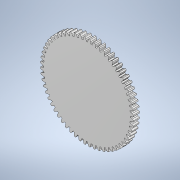
# Autodesk Inventor part: 二段m1z60
Saved by Autodesk Inventor 2022.2 (Build 262287010, 287A)
## iProperties
Created: 2022-03-13
Part Number: 二段m1z60
Material: Aluminum 2014-T6
Document SubType Name: Modeling
Designer: acps
Density: 2.78927 g/cm^3
Appearance: Satin
Author: acps
Autodesk Inventor part; units mm, degrees
ref_plane "YZ Plane" through (0, 0, 0) normal (1, 0, 0) x (0, 1, 0)
ref_plane "XZ Plane" through (0, 0, 0) normal (0, 1, 0) x (-1, 0, 0)
ref_plane "XY Plane" through (0, 0, 0) normal (0, 0, 1) x (1, 0, 0)
sketch "Sketch1" plane through (0, 0, 0) normal (0, 0, 1) x (1, 0, 0)
  arc A0 (0.5381, 29.2813) -> (0.3992, 28.7472) centre (7.046, 27.304) ccw
  arc A1 (0.7944, 30.0128) -> (0.5381, 29.2813) centre (9.2841, 26.6271) ccw
  arc A2 (1.223, 30.9617) -> (0.7944, 30.0128) centre (11.5695, 25.7177) ccw
  arc A3 (-2.5272, 29.1688) -> (-2.6079, 28.6315) centre (4.1534, 27.891) ccw
  arc A4 (-2.3471, 29.9314) -> (-2.5272, 29.1688) centre (6.45, 27.4517) ccw
  arc A5 (-2.0201, 30.9199) -> (-2.3471, 29.9314) centre (8.8179, 26.7861) ccw
  arc A6 (-5.5616, 28.7533) -> (-5.5864, 28.202) centre (1.2152, 28.1723) ccw
  arc A7 (-5.4629, 29.5221) -> (-5.5616, 28.7533) centre (3.5452, 27.9755) ccw
  arc A8 (-5.241, 30.5394) -> (-5.4629, 29.5221) centre (5.9697, 27.5611) ccw
  arc A9 (-8.5367, 28.0144) -> (-8.5037, 27.4636) centre (-1.7362, 28.145) ccw
  arc A10 (-8.5189, 28.7893) -> (-8.5367, 28.0144) centre (0.6015, 28.1928) ccw
  arc A11 (-8.4046, 29.8243) -> (-8.5189, 28.7893) centre (3.0561, 28.0342) ccw
  arc A12 (-11.4182, 26.9686) -> (-11.3278, 26.4243) centre (-4.6687, 27.8093) ccw
  arc A13 (-11.4816, 27.7412) -> (-11.4182, 26.9686) centre (-2.3488, 28.1012) ccw
  arc A14 (-11.476, 28.7824) -> (-11.4816, 27.7412) centre (0.109, 28.2) ccw
  arc A15 (-14.1746, 25.6274) -> (-14.0279, 25.0954) centre (-7.55, 27.169) ccw
  arc A16 (-14.3184, 26.389) -> (-14.1746, 25.6274) centre (-5.2733, 27.7018) ccw
  arc A17 (-14.4217, 27.4251) -> (-14.3184, 26.389) centre (-2.8393, 28.057) ccw
  arc A18 (-16.7758, 24.0053) -> (-16.5742, 23.4917) centre (-10.3486, 26.231) ccw
  arc A19 (-16.9984, 24.7478) -> (-16.7758, 24.0053) centre (-8.14, 26.9988) ccw
  arc A20 (-17.2094, 25.7674) -> (-16.9984, 24.7478) centre (-5.7565, 27.6065) ccw
  arc A21 (-19.1931, 22.1203) -> (-18.939, 21.6305) centre (-13.0337, 25.0056) ccw
  arc A22 (-19.4921, 22.8354) -> (-19.1931, 22.1203) centre (-10.9176, 26.0001) ccw
  arc A23 (-19.8086, 23.8274) -> (-19.4921, 22.8354) centre (-8.6106, 26.8535) ccw
  arc A24 (-21.4002, 19.9929) -> (-21.0962, 19.5323) centre (-15.5761, 23.5062) ccw
  arc A25 (-21.7723, 20.6728) -> (-21.4002, 19.9929) centre (-13.5755, 24.7164) ccw
  arc A26 (-22.1907, 21.6263) -> (-21.7723, 20.6728) centre (-11.3704, 25.8063) ccw
  arc A27 (-23.3728, 17.6464) -> (-23.0223, 17.2202) centre (-17.9479, 21.7493) ccw
  arc A28 (-23.8139, 18.2838) -> (-23.3728, 17.6464) centre (-16.0847, 23.162) ccw
  arc A29 (-24.3297, 19.1883) -> (-23.8139, 18.2838) centre (-14.0056, 24.4764) ccw
  arc A30 (-25.0893, 15.1066) -> (-24.6962, 14.7194) centre (-20.123, 19.754) ccw
  arc A31 (-25.5946, 15.6944) -> (-25.0893, 15.1066) centre (-18.4177, 21.3538) ccw
  arc A32 (-26.2021, 16.54) -> (-25.5946, 15.6944) centre (-16.4874, 22.8784) ccw
  arc A33 (-26.5309, 12.4013) -> (-26.0995, 12.0573) centre (-22.0776, 17.5424) ccw
  arc A34 (-27.0949, 12.933) -> (-26.5309, 12.4013) centre (-20.5489, 19.3117) ccw
  arc A35 (-27.7875, 13.7105) -> (-27.0949, 12.933) centre (-18.7885, 21.0296) ccw
  arc A36 (-27.6819, 9.5602) -> (-27.2169, 9.2631) centre (-23.7903, 15.1386) ccw
  arc A37 (-28.2984, 10.03) -> (-27.6819, 9.5602) centre (-22.4549, 17.0579) ccw
  arc A38 (-29.0684, 10.7308) -> (-28.2984, 10.03) centre (-20.8838, 18.9505) ccw
  arc A39 (-28.5295, 6.6143) -> (-28.036, 6.3674) centre (-25.2424, 12.5689) ccw
  arc A40 (-29.1918, 7.0171) -> (-28.5295, 6.6143) centre (-24.1149, 14.6173) ccw
  arc A41 (-30.0309, 7.6336) -> (-29.1918, 7.0171) centre (-22.7503, 16.6637) ccw
  arc A42 (-29.0646, 3.5959) -> (-28.548, 3.4019) centre (-26.4179, 9.8615) ccw
  arc A43 (-29.7653, 3.9273) -> (-29.0646, 3.5959) centre (-25.5108, 12.0165) ccw
  arc A44 (-30.6643, 4.4527) -> (-29.7653, 3.9273) centre (-24.3675, 14.1944) ccw
  arc A45 (-29.2813, 0.5381) -> (-28.7472, 0.3992) centre (-27.304, 7.046) ccw
  arc A46 (-30.0128, 0.7944) -> (-29.2813, 0.5381) centre (-26.6271, 9.2841) ccw
  arc A47 (-30.9617, 1.223) -> (-30.0128, 0.7944) centre (-25.7177, 11.5695) ccw
  arc A48 (-29.1771, -2.5256) -> (-28.6315, -2.6079) centre (-27.891, 4.1534) ccw
  arc A49 (-29.9314, -2.3471) -> (-29.1771, -2.5256) centre (-27.4517, 6.45) ccw
  arc A50 (-30.9199, -2.0201) -> (-29.9314, -2.3471) centre (-26.7862, 8.8179) ccw
  arc A51 (-28.7533, -5.5616) -> (-28.202, -5.5864) centre (-28.1723, 1.2152) ccw
  arc A52 (-29.5221, -5.4629) -> (-28.7533, -5.5616) centre (-27.9755, 3.5452) ccw
  arc A53 (-30.5394, -5.241) -> (-29.5221, -5.4629) centre (-27.5611, 5.9697) ccw
  arc A54 (-28.0144, -8.5367) -> (-27.4636, -8.5037) centre (-28.145, -1.7362) ccw
  arc A55 (-28.7893, -8.5189) -> (-28.0144, -8.5367) centre (-28.1928, 0.6015) ccw
  arc A56 (-29.8243, -8.4046) -> (-28.7893, -8.5189) centre (-28.0342, 3.0561) ccw
  arc A57 (-26.9686, -11.4182) -> (-26.4243, -11.3278) centre (-27.8093, -4.6687) ccw
  arc A58 (-27.7412, -11.4816) -> (-26.9686, -11.4182) centre (-28.1012, -2.3488) ccw
  arc A59 (-28.7824, -11.476) -> (-27.7412, -11.4816) centre (-28.2, 0.109) ccw
  arc A60 (-25.6274, -14.1746) -> (-25.0954, -14.0279) centre (-27.169, -7.55) ccw
  arc A61 (-26.389, -14.3184) -> (-25.6274, -14.1746) centre (-27.7018, -5.2733) ccw
  arc A62 (-27.4251, -14.4217) -> (-26.389, -14.3184) centre (-28.057, -2.8393) ccw
  arc A63 (-24.0053, -16.7758) -> (-23.4917, -16.5742) centre (-26.231, -10.3486) ccw
  arc A64 (-24.741, -16.9966) -> (-24.0053, -16.7758) centre (-26.9988, -8.14) ccw
  arc A65 (-25.7674, -17.2094) -> (-24.741, -16.9966) centre (-27.6065, -5.7565) ccw
  arc A66 (-22.1126, -19.1895) -> (-21.6305, -18.939) centre (-25.0056, -13.0337) ccw
  arc A67 (-22.8354, -19.4921) -> (-22.1126, -19.1895) centre (-26.0001, -10.9176) ccw
  arc A68 (-23.8274, -19.8086) -> (-22.8354, -19.4921) centre (-26.8535, -8.6106) ccw
  arc A69 (-19.9929, -21.4002) -> (-19.5323, -21.0962) centre (-23.5062, -15.5761) ccw
  arc A70 (-20.6728, -21.7723) -> (-19.9929, -21.4002) centre (-24.7164, -13.5755) ccw
  arc A71 (-21.6263, -22.1907) -> (-20.6728, -21.7723) centre (-25.8063, -11.3704) ccw
  arc A72 (-17.6464, -23.3728) -> (-17.2202, -23.0223) centre (-21.7493, -17.9479) ccw
  arc A73 (-18.2838, -23.8139) -> (-17.6464, -23.3728) centre (-23.162, -16.0847) ccw
  arc A74 (-19.1883, -24.3297) -> (-18.2838, -23.8139) centre (-24.4764, -14.0056) ccw
  arc A75 (-15.1066, -25.0893) -> (-14.7194, -24.6962) centre (-19.754, -20.123) ccw
  arc A76 (-15.6944, -25.5946) -> (-15.1066, -25.0893) centre (-21.3538, -18.4177) ccw
  arc A77 (-16.54, -26.2021) -> (-15.6944, -25.5946) centre (-22.8784, -16.4874) ccw
  arc A78 (-12.4013, -26.5309) -> (-12.0573, -26.0995) centre (-17.5424, -22.0776) ccw
  arc A79 (-12.933, -27.0949) -> (-12.4013, -26.5309) centre (-19.3117, -20.5489) ccw
  arc A80 (-13.7105, -27.7875) -> (-12.933, -27.0949) centre (-21.0296, -18.7885) ccw
  arc A81 (-9.5602, -27.6819) -> (-9.2631, -27.2169) centre (-15.1386, -23.7903) ccw
  arc A82 (-10.03, -28.2984) -> (-9.5602, -27.6819) centre (-17.0579, -22.4549) ccw
  arc A83 (-10.7308, -29.0684) -> (-10.03, -28.2984) centre (-18.9505, -20.8838) ccw
  arc A84 (-6.6143, -28.5295) -> (-6.3674, -28.036) centre (-12.5689, -25.2424) ccw
  arc A85 (-7.0171, -29.1918) -> (-6.6143, -28.5295) centre (-14.6173, -24.1149) ccw
  arc A86 (-7.6336, -30.0309) -> (-7.0171, -29.1918) centre (-16.6637, -22.7503) ccw
  arc A87 (-3.5959, -29.0646) -> (-3.4019, -28.548) centre (-9.8615, -26.4179) ccw
  arc A88 (-3.9273, -29.7653) -> (-3.5959, -29.0646) centre (-12.0165, -25.5108) ccw
  arc A89 (-4.4527, -30.6643) -> (-3.9273, -29.7653) centre (-14.1944, -24.3675) ccw
  arc A90 (-0.5381, -29.2813) -> (-0.3992, -28.7472) centre (-7.046, -27.304) ccw
  arc A91 (-0.7944, -30.0128) -> (-0.5381, -29.2813) centre (-9.2841, -26.6271) ccw
  arc A92 (-1.223, -30.9617) -> (-0.7944, -30.0128) centre (-11.5695, -25.7177) ccw
  arc A93 (2.5256, -29.1771) -> (2.6079, -28.6315) centre (-4.1534, -27.891) ccw
  arc A94 (2.3471, -29.9314) -> (2.5256, -29.1771) centre (-6.45, -27.4517) ccw
  arc A95 (2.0201, -30.9199) -> (2.3471, -29.9314) centre (-8.8179, -26.7862) ccw
  arc A96 (5.5616, -28.7533) -> (5.5864, -28.202) centre (-1.2152, -28.1723) ccw
  arc A97 (5.4629, -29.5221) -> (5.5616, -28.7533) centre (-3.5452, -27.9755) ccw
  arc A98 (5.241, -30.5394) -> (5.4629, -29.5221) centre (-5.9697, -27.5611) ccw
  arc A99 (8.5367, -28.0144) -> (8.5037, -27.4636) centre (1.7362, -28.145) ccw
  arc A100 (8.5189, -28.7893) -> (8.5367, -28.0144) centre (-0.6015, -28.1928) ccw
  arc A101 (8.4046, -29.8243) -> (8.5189, -28.7893) centre (-3.0561, -28.0342) ccw
  arc A102 (11.4182, -26.9686) -> (11.3278, -26.4243) centre (4.6687, -27.8093) ccw
  arc A103 (11.4816, -27.7412) -> (11.4182, -26.9686) centre (2.3488, -28.1012) ccw
  arc A104 (11.476, -28.7824) -> (11.4816, -27.7412) centre (-0.109, -28.2) ccw
  arc A105 (14.1746, -25.6274) -> (14.0279, -25.0954) centre (7.55, -27.169) ccw
  arc A106 (14.3184, -26.389) -> (14.1746, -25.6274) centre (5.2733, -27.7018) ccw
  arc A107 (14.4217, -27.4251) -> (14.3184, -26.389) centre (2.8393, -28.057) ccw
  arc A108 (16.7758, -24.0053) -> (16.5742, -23.4917) centre (10.3486, -26.231) ccw
  arc A109 (16.9984, -24.7478) -> (16.7758, -24.0053) centre (8.14, -26.9988) ccw
  arc A110 (17.2094, -25.7674) -> (16.9984, -24.7478) centre (5.7565, -27.6065) ccw
  arc A111 (19.1931, -22.1203) -> (18.939, -21.6305) centre (13.0337, -25.0056) ccw
  arc A112 (19.4921, -22.8354) -> (19.1931, -22.1203) centre (10.9176, -26.0001) ccw
  arc A113 (19.8086, -23.8274) -> (19.4921, -22.8354) centre (8.6106, -26.8535) ccw
  arc A114 (21.4002, -19.9929) -> (21.0962, -19.5323) centre (15.5761, -23.5062) ccw
  arc A115 (21.7723, -20.6728) -> (21.4002, -19.9929) centre (13.5755, -24.7164) ccw
  arc A116 (22.1907, -21.6263) -> (21.7723, -20.6728) centre (11.3704, -25.8063) ccw
  arc A117 (23.3728, -17.6464) -> (23.0223, -17.2202) centre (17.9479, -21.7493) ccw
  arc A118 (23.8139, -18.2838) -> (23.3728, -17.6464) centre (16.0847, -23.162) ccw
  arc A119 (24.3297, -19.1883) -> (23.8139, -18.2838) centre (14.0056, -24.4764) ccw
  arc A120 (25.0893, -15.1066) -> (24.6962, -14.7194) centre (20.123, -19.754) ccw
  arc A121 (25.5946, -15.6944) -> (25.0893, -15.1066) centre (18.4177, -21.3538) ccw
  arc A122 (26.2021, -16.54) -> (25.5946, -15.6944) centre (16.4874, -22.8784) ccw
  arc A123 (26.5309, -12.4013) -> (26.0995, -12.0573) centre (22.0776, -17.5424) ccw
  arc A124 (27.0949, -12.933) -> (26.5309, -12.4013) centre (20.5489, -19.3117) ccw
  arc A125 (27.7875, -13.7105) -> (27.0949, -12.933) centre (18.7885, -21.0296) ccw
  arc A126 (27.6819, -9.5602) -> (27.2169, -9.2631) centre (23.7903, -15.1386) ccw
  arc A127 (28.2984, -10.03) -> (27.6819, -9.5602) centre (22.4549, -17.0579) ccw
  arc A128 (29.0684, -10.7308) -> (28.2984, -10.03) centre (20.8838, -18.9505) ccw
  arc A129 (28.5295, -6.6143) -> (28.036, -6.3674) centre (25.2424, -12.5689) ccw
  arc A130 (29.1918, -7.0171) -> (28.5295, -6.6143) centre (24.1149, -14.6173) ccw
  arc A131 (30.0309, -7.6336) -> (29.1918, -7.0171) centre (22.7503, -16.6637) ccw
  arc A132 (29.0646, -3.5959) -> (28.548, -3.4019) centre (26.4179, -9.8615) ccw
  arc A133 (29.7653, -3.9273) -> (29.0646, -3.5959) centre (25.5108, -12.0165) ccw
  arc A134 (30.6643, -4.4527) -> (29.7653, -3.9273) centre (24.3675, -14.1944) ccw
  arc A135 (29.2813, -0.5381) -> (28.7472, -0.3992) centre (27.304, -7.046) ccw
  arc A136 (30.0128, -0.7944) -> (29.2813, -0.5381) centre (26.6271, -9.2841) ccw
  arc A137 (30.9617, -1.223) -> (30.0128, -0.7944) centre (25.7177, -11.5695) ccw
  arc A138 (29.1771, 2.5256) -> (28.6315, 2.6079) centre (27.891, -4.1534) ccw
  arc A139 (29.9314, 2.3471) -> (29.1771, 2.5256) centre (27.4517, -6.45) ccw
  arc A140 (30.9199, 2.0201) -> (29.9314, 2.3471) centre (26.7862, -8.8179) ccw
  arc A141 (28.7533, 5.5616) -> (28.202, 5.5864) centre (28.1723, -1.2152) ccw
  arc A142 (29.5221, 5.4629) -> (28.7533, 5.5616) centre (27.9755, -3.5452) ccw
  arc A143 (30.5394, 5.241) -> (29.5221, 5.4629) centre (27.5611, -5.9697) ccw
  arc A144 (28.0144, 8.5367) -> (27.4636, 8.5037) centre (28.145, 1.7362) ccw
  arc A145 (28.7893, 8.5189) -> (28.0144, 8.5367) centre (28.1928, -0.6015) ccw
  arc A146 (29.8243, 8.4046) -> (28.7893, 8.5189) centre (28.0342, -3.0561) ccw
  arc A147 (26.9686, 11.4182) -> (26.4243, 11.3278) centre (27.8093, 4.6687) ccw
  arc A148 (27.7412, 11.4816) -> (26.9686, 11.4182) centre (28.1012, 2.3488) ccw
  arc A149 (28.7824, 11.476) -> (27.7412, 11.4816) centre (28.2, -0.109) ccw
  arc A150 (25.6274, 14.1746) -> (25.0954, 14.0279) centre (27.169, 7.55) ccw
  arc A151 (26.389, 14.3184) -> (25.6274, 14.1746) centre (27.7018, 5.2733) ccw
  arc A152 (27.4251, 14.4217) -> (26.389, 14.3184) centre (28.057, 2.8393) ccw
  arc A153 (24.0053, 16.7758) -> (23.4917, 16.5742) centre (26.231, 10.3486) ccw
  arc A154 (24.7478, 16.9984) -> (24.0053, 16.7758) centre (26.9988, 8.14) ccw
  arc A155 (25.7674, 17.2094) -> (24.7478, 16.9984) centre (27.6065, 5.7565) ccw
  arc A156 (22.1203, 19.1931) -> (21.6305, 18.939) centre (25.0056, 13.0337) ccw
  arc A157 (22.8354, 19.4921) -> (22.1203, 19.1931) centre (26.0001, 10.9176) ccw
  arc A158 (23.8274, 19.8086) -> (22.8354, 19.4921) centre (26.8535, 8.6106) ccw
  arc A159 (19.9929, 21.4002) -> (19.5323, 21.0962) centre (23.5062, 15.5761) ccw
  arc A160 (20.6728, 21.7723) -> (19.9929, 21.4002) centre (24.7164, 13.5755) ccw
  arc A161 (21.6263, 22.1907) -> (20.6728, 21.7723) centre (25.8063, 11.3704) ccw
  arc A162 (17.6464, 23.3728) -> (17.2202, 23.0223) centre (21.7493, 17.9479) ccw
  arc A163 (18.2838, 23.8139) -> (17.6464, 23.3728) centre (23.162, 16.0847) ccw
  arc A164 (19.1883, 24.3297) -> (18.2838, 23.8139) centre (24.4764, 14.0056) ccw
  arc A165 (15.1066, 25.0893) -> (14.7194, 24.6962) centre (19.754, 20.123) ccw
  arc A166 (15.6944, 25.5946) -> (15.1066, 25.0893) centre (21.3538, 18.4177) ccw
  arc A167 (16.54, 26.2021) -> (15.6944, 25.5946) centre (22.8784, 16.4874) ccw
  arc A168 (12.4013, 26.5309) -> (12.0573, 26.0995) centre (17.5424, 22.0776) ccw
  arc A169 (12.933, 27.0949) -> (12.4013, 26.5309) centre (19.3117, 20.5489) ccw
  arc A170 (13.7105, 27.7875) -> (12.933, 27.0949) centre (21.0296, 18.7885) ccw
  arc A171 (9.5602, 27.6819) -> (9.2631, 27.2169) centre (15.1386, 23.7903) ccw
  arc A172 (10.03, 28.2984) -> (9.5602, 27.6819) centre (17.0579, 22.4549) ccw
  arc A173 (10.7308, 29.0684) -> (10.03, 28.2984) centre (18.9505, 20.8838) ccw
  arc A174 (6.6143, 28.5295) -> (6.3674, 28.036) centre (12.5689, 25.2424) ccw
  arc A175 (7.0171, 29.1918) -> (6.6143, 28.5295) centre (14.6173, 24.1149) ccw
  arc A176 (7.6336, 30.0309) -> (7.0171, 29.1918) centre (16.6637, 22.7503) ccw
  arc A177 (3.5959, 29.0646) -> (3.4019, 28.548) centre (9.8615, 26.4179) ccw
  arc A178 (3.9273, 29.7653) -> (3.5959, 29.0646) centre (12.0165, 25.5108) ccw
  arc A179 (4.4527, 30.6643) -> (3.9273, 29.7653) centre (14.1944, 24.3675) ccw
  arc A180 (-0.3992, 28.7472) -> (-0.5381, 29.2813) centre (-7.046, 27.304) ccw
  arc A181 (-0.5381, 29.2813) -> (-0.7944, 30.0128) centre (-9.2841, 26.6271) ccw
  arc A182 (-0.7944, 30.0128) -> (-1.223, 30.9617) centre (-11.5695, 25.7177) ccw
  arc A183 (-3.4019, 28.548) -> (-3.5959, 29.0646) centre (-9.8615, 26.4179) ccw
  arc A184 (-3.5959, 29.0646) -> (-3.9273, 29.7653) centre (-12.0165, 25.5108) ccw
  arc A185 (-3.9273, 29.7653) -> (-4.4527, 30.6643) centre (-14.1944, 24.3675) ccw
  arc A186 (-6.3674, 28.036) -> (-6.6143, 28.5295) centre (-12.5689, 25.2424) ccw
  arc A187 (-6.6143, 28.5295) -> (-7.0171, 29.1918) centre (-14.6173, 24.1149) ccw
  arc A188 (-7.0171, 29.1918) -> (-7.6336, 30.0309) centre (-16.6637, 22.7503) ccw
  arc A189 (-9.2631, 27.2169) -> (-9.5602, 27.6819) centre (-15.1386, 23.7903) ccw
  arc A190 (-9.5602, 27.6819) -> (-10.03, 28.2984) centre (-17.0579, 22.4549) ccw
  arc A191 (-10.03, 28.2984) -> (-10.7308, 29.0684) centre (-18.9505, 20.8838) ccw
  arc A192 (-12.0573, 26.0995) -> (-12.4013, 26.5309) centre (-17.5424, 22.0776) ccw
  arc A193 (-12.4013, 26.5309) -> (-12.933, 27.0949) centre (-19.3117, 20.5489) ccw
  arc A194 (-12.933, 27.0949) -> (-13.7105, 27.7875) centre (-21.0296, 18.7885) ccw
  arc A195 (-14.7194, 24.6962) -> (-15.1066, 25.0893) centre (-19.754, 20.123) ccw
  arc A196 (-15.1066, 25.0893) -> (-15.6944, 25.5946) centre (-21.3538, 18.4177) ccw
  arc A197 (-15.6944, 25.5946) -> (-16.54, 26.2021) centre (-22.8784, 16.4874) ccw
  arc A198 (-17.2202, 23.0223) -> (-17.6464, 23.3728) centre (-21.7493, 17.9479) ccw
  arc A199 (-17.6464, 23.3728) -> (-18.2838, 23.8139) centre (-23.162, 16.0847) ccw
  arc A200 (-18.2838, 23.8139) -> (-19.1883, 24.3297) centre (-24.4764, 14.0056) ccw
  arc A201 (-19.5323, 21.0962) -> (-19.9929, 21.4002) centre (-23.5062, 15.5761) ccw
  arc A202 (-19.9929, 21.4002) -> (-20.6728, 21.7723) centre (-24.7164, 13.5755) ccw
  arc A203 (-20.6728, 21.7723) -> (-21.6263, 22.1907) centre (-25.8063, 11.3704) ccw
  arc A204 (-21.6305, 18.939) -> (-22.1203, 19.1931) centre (-25.0056, 13.0337) ccw
  arc A205 (-22.1203, 19.1931) -> (-22.8354, 19.4921) centre (-26.0001, 10.9176) ccw
  arc A206 (-22.8354, 19.4921) -> (-23.8274, 19.8086) centre (-26.8535, 8.6106) ccw
  arc A207 (-23.4917, 16.5742) -> (-24.0053, 16.7758) centre (-26.231, 10.3486) ccw
  arc A208 (-24.0053, 16.7758) -> (-24.7478, 16.9984) centre (-26.9988, 8.14) ccw
  arc A209 (-24.7478, 16.9984) -> (-25.7674, 17.2094) centre (-27.6065, 5.7565) ccw
  arc A210 (-25.0954, 14.0279) -> (-25.6274, 14.1746) centre (-27.169, 7.55) ccw
  arc A211 (-25.6274, 14.1746) -> (-26.389, 14.3184) centre (-27.7018, 5.2733) ccw
  arc A212 (-26.389, 14.3184) -> (-27.4251, 14.4217) centre (-28.057, 2.8393) ccw
  arc A213 (-26.4243, 11.3278) -> (-26.9686, 11.4182) centre (-27.8093, 4.6687) ccw
  arc A214 (-26.9686, 11.4182) -> (-27.7412, 11.4816) centre (-28.1012, 2.3488) ccw
  arc A215 (-27.7412, 11.4816) -> (-28.7824, 11.476) centre (-28.2, -0.109) ccw
  arc A216 (-27.4636, 8.5037) -> (-28.0144, 8.5367) centre (-28.145, 1.7362) ccw
  arc A217 (-28.0144, 8.5367) -> (-28.7893, 8.5189) centre (-28.1928, -0.6015) ccw
  arc A218 (-28.7893, 8.5189) -> (-29.8243, 8.4046) centre (-28.0342, -3.0561) ccw
  arc A219 (-28.202, 5.5864) -> (-28.7533, 5.5616) centre (-28.1723, -1.2152) ccw
  arc A220 (-28.7533, 5.5616) -> (-29.5221, 5.4629) centre (-27.9755, -3.5452) ccw
  arc A221 (-29.5221, 5.4629) -> (-30.5394, 5.241) centre (-27.5611, -5.9697) ccw
  arc A222 (-28.6315, 2.6079) -> (-29.1771, 2.5256) centre (-27.891, -4.1534) ccw
  arc A223 (-29.1771, 2.5256) -> (-29.9314, 2.3471) centre (-27.4517, -6.45) ccw
  arc A224 (-29.9314, 2.3471) -> (-30.9199, 2.0201) centre (-26.7862, -8.8179) ccw
  arc A225 (-28.7472, -0.3992) -> (-29.2813, -0.5381) centre (-27.304, -7.046) ccw
  arc A226 (-29.2813, -0.5381) -> (-30.0128, -0.7944) centre (-26.6271, -9.2841) ccw
  arc A227 (-30.0128, -0.7944) -> (-30.9617, -1.223) centre (-25.7177, -11.5695) ccw
  arc A228 (-28.548, -3.4019) -> (-29.0646, -3.5959) centre (-26.4179, -9.8615) ccw
  arc A229 (-29.0646, -3.5959) -> (-29.7653, -3.9273) centre (-25.5108, -12.0165) ccw
  arc A230 (-29.7653, -3.9273) -> (-30.6643, -4.4527) centre (-24.3675, -14.1944) ccw
  arc A231 (-28.036, -6.3674) -> (-28.5295, -6.6143) centre (-25.2424, -12.5689) ccw
  arc A232 (-28.5295, -6.6143) -> (-29.1918, -7.0171) centre (-24.1149, -14.6173) ccw
  arc A233 (-29.1918, -7.0171) -> (-30.0309, -7.6336) centre (-22.7503, -16.6637) ccw
  arc A234 (-27.2169, -9.2631) -> (-27.6819, -9.5602) centre (-23.7903, -15.1386) ccw
  arc A235 (-27.6819, -9.5602) -> (-28.2984, -10.03) centre (-22.4549, -17.0579) ccw
  arc A236 (-28.2984, -10.03) -> (-29.0684, -10.7308) centre (-20.8838, -18.9505) ccw
  arc A237 (-26.0995, -12.0573) -> (-26.5309, -12.4013) centre (-22.0776, -17.5424) ccw
  arc A238 (-26.5309, -12.4013) -> (-27.0949, -12.933) centre (-20.5489, -19.3117) ccw
  arc A239 (-27.0949, -12.933) -> (-27.7875, -13.7105) centre (-18.7885, -21.0296) ccw
  arc A240 (-24.6962, -14.7194) -> (-25.0893, -15.1066) centre (-20.123, -19.754) ccw
  arc A241 (-25.0893, -15.1066) -> (-25.5946, -15.6944) centre (-18.4177, -21.3538) ccw
  arc A242 (-25.5946, -15.6944) -> (-26.2021, -16.54) centre (-16.4874, -22.8784) ccw
  arc A243 (-23.0223, -17.2202) -> (-23.3728, -17.6464) centre (-17.9479, -21.7493) ccw
  arc A244 (-23.3728, -17.6464) -> (-23.8139, -18.2838) centre (-16.0847, -23.162) ccw
  arc A245 (-23.8139, -18.2838) -> (-24.3297, -19.1883) centre (-14.0056, -24.4764) ccw
  arc A246 (-21.0962, -19.5323) -> (-21.4002, -19.9929) centre (-15.5761, -23.5062) ccw
  arc A247 (-21.4002, -19.9929) -> (-21.7723, -20.6728) centre (-13.5755, -24.7164) ccw
  arc A248 (-21.7723, -20.6728) -> (-22.1907, -21.6263) centre (-11.3704, -25.8063) ccw
  arc A249 (-18.939, -21.6305) -> (-19.1931, -22.1203) centre (-13.0337, -25.0056) ccw
  arc A250 (-19.1931, -22.1203) -> (-19.4921, -22.8354) centre (-10.9176, -26.0001) ccw
  arc A251 (-19.4921, -22.8354) -> (-19.8086, -23.8274) centre (-8.6106, -26.8535) ccw
  arc A252 (-16.5742, -23.4917) -> (-16.7758, -24.0053) centre (-10.3486, -26.231) ccw
  arc A253 (-16.7758, -24.0053) -> (-16.9984, -24.7478) centre (-8.14, -26.9988) ccw
  arc A254 (-16.9984, -24.7478) -> (-17.2094, -25.7674) centre (-5.7565, -27.6065) ccw
  arc A255 (-14.0279, -25.0954) -> (-14.1746, -25.6274) centre (-7.55, -27.169) ccw
  arc A256 (-14.1746, -25.6274) -> (-14.3184, -26.389) centre (-5.2733, -27.7018) ccw
  arc A257 (-14.3184, -26.389) -> (-14.4217, -27.4251) centre (-2.8393, -28.0569) ccw
  arc A258 (-11.3278, -26.4243) -> (-11.4182, -26.9686) centre (-4.6687, -27.8093) ccw
  arc A259 (-11.4182, -26.9686) -> (-11.4816, -27.7411) centre (-2.3488, -28.1012) ccw
  arc A260 (-11.4816, -27.7411) -> (-11.476, -28.7824) centre (0.109, -28.2) ccw
  arc A261 (-8.5037, -27.4636) -> (-8.5367, -28.0144) centre (-1.7362, -28.145) ccw
  arc A262 (-8.5367, -28.0144) -> (-8.5189, -28.7893) centre (0.6015, -28.1928) ccw
  arc A263 (-8.5189, -28.7893) -> (-8.4046, -29.8243) centre (3.0561, -28.0342) ccw
  arc A264 (-5.5864, -28.202) -> (-5.5616, -28.7533) centre (1.2152, -28.1723) ccw
  arc A265 (-5.5616, -28.7533) -> (-5.4629, -29.5221) centre (3.5452, -27.9755) ccw
  arc A266 (-5.4629, -29.5221) -> (-5.241, -30.5394) centre (5.9697, -27.5611) ccw
  arc A267 (-2.6079, -28.6315) -> (-2.5256, -29.1771) centre (4.1534, -27.891) ccw
  arc A268 (-2.5256, -29.1771) -> (-2.3471, -29.9314) centre (6.45, -27.4517) ccw
  arc A269 (-2.3471, -29.9314) -> (-2.0201, -30.9199) centre (8.8179, -26.7862) ccw
  arc A270 (0.3992, -28.7472) -> (0.5356, -29.2732) centre (7.046, -27.304) ccw
  arc A271 (0.5356, -29.2732) -> (0.7944, -30.0128) centre (9.2841, -26.6271) ccw
  arc A272 (0.7944, -30.0128) -> (1.223, -30.9617) centre (11.5695, -25.7177) ccw
  arc A273 (3.4019, -28.548) -> (3.5959, -29.0646) centre (9.8615, -26.4179) ccw
  arc A274 (3.5959, -29.0646) -> (3.924, -29.7591) centre (12.0165, -25.5108) ccw
  arc A275 (3.924, -29.7591) -> (4.4527, -30.6643) centre (14.1944, -24.3675) ccw
  arc A276 (6.3674, -28.036) -> (6.6143, -28.5295) centre (12.5689, -25.2424) ccw
  arc A277 (6.6143, -28.5295) -> (7.0171, -29.1918) centre (14.6173, -24.1149) ccw
  arc A278 (7.0171, -29.1918) -> (7.6336, -30.0309) centre (16.6637, -22.7503) ccw
  arc A279 (9.2631, -27.2169) -> (9.5553, -27.6749) centre (15.1386, -23.7903) ccw
  arc A280 (9.5553, -27.6749) -> (10.03, -28.2984) centre (17.0579, -22.4549) ccw
  arc A281 (10.03, -28.2984) -> (10.7308, -29.0684) centre (18.9505, -20.8838) ccw
  arc A282 (12.0573, -26.0995) -> (12.4013, -26.5309) centre (17.5424, -22.0776) ccw
  arc A283 (12.4013, -26.5309) -> (12.933, -27.0949) centre (19.3117, -20.5489) ccw
  arc A284 (12.933, -27.0949) -> (13.7105, -27.7875) centre (21.0296, -18.7885) ccw
  arc A285 (14.7194, -24.6962) -> (15.1066, -25.0893) centre (19.754, -20.123) ccw
  arc A286 (15.1066, -25.0893) -> (15.6944, -25.5946) centre (21.3538, -18.4177) ccw
  arc A287 (15.6944, -25.5946) -> (16.54, -26.2021) centre (22.8784, -16.4874) ccw
  arc A288 (17.2202, -23.0223) -> (17.6464, -23.3728) centre (21.7493, -17.9479) ccw
  arc A289 (17.6464, -23.3728) -> (18.2838, -23.8139) centre (23.162, -16.0847) ccw
  arc A290 (18.2838, -23.8139) -> (19.1883, -24.3297) centre (24.4764, -14.0056) ccw
  arc A291 (19.5323, -21.0962) -> (19.9929, -21.4002) centre (23.5062, -15.5761) ccw
  arc A292 (19.9929, -21.4002) -> (20.6728, -21.7723) centre (24.7164, -13.5755) ccw
  arc A293 (20.6728, -21.7723) -> (21.6263, -22.1907) centre (25.8063, -11.3704) ccw
  arc A294 (21.6305, -18.939) -> (22.1203, -19.1931) centre (25.0056, -13.0337) ccw
  arc A295 (22.1203, -19.1931) -> (22.8354, -19.4921) centre (26.0001, -10.9176) ccw
  arc A296 (22.8354, -19.4921) -> (23.8274, -19.8086) centre (26.8535, -8.6106) ccw
  arc A297 (23.4917, -16.5742) -> (24.0053, -16.7758) centre (26.231, -10.3486) ccw
  arc A298 (24.0053, -16.7758) -> (24.7478, -16.9984) centre (26.9988, -8.14) ccw
  arc A299 (24.7478, -16.9984) -> (25.7674, -17.2094) centre (27.6065, -5.7565) ccw
  arc A300 (25.0954, -14.0279) -> (25.6274, -14.1746) centre (27.169, -7.55) ccw
  arc A301 (25.6274, -14.1746) -> (26.389, -14.3184) centre (27.7018, -5.2733) ccw
  arc A302 (26.389, -14.3184) -> (27.4251, -14.4217) centre (28.057, -2.8393) ccw
  arc A303 (26.4243, -11.3278) -> (26.9686, -11.4182) centre (27.8093, -4.6687) ccw
  arc A304 (26.9686, -11.4182) -> (27.7412, -11.4816) centre (28.1012, -2.3488) ccw
  arc A305 (27.7412, -11.4816) -> (28.7824, -11.476) centre (28.2, 0.109) ccw
  arc A306 (27.4636, -8.5037) -> (28.006, -8.5365) centre (28.145, -1.7362) ccw
  arc A307 (28.006, -8.5365) -> (28.7893, -8.5189) centre (28.1928, 0.6015) ccw
  arc A308 (28.7893, -8.5189) -> (29.8243, -8.4046) centre (28.0342, 3.0561) ccw
  arc A309 (28.202, -5.5864) -> (28.7533, -5.5616) centre (28.1723, 1.2152) ccw
  arc A310 (28.7533, -5.5616) -> (29.5221, -5.4629) centre (27.9755, 3.5452) ccw
  arc A311 (29.5221, -5.4629) -> (30.5394, -5.241) centre (27.5611, 5.9697) ccw
  arc A312 (28.6315, -2.6079) -> (29.1771, -2.5256) centre (27.891, 4.1534) ccw
  arc A313 (29.1771, -2.5256) -> (29.9314, -2.3471) centre (27.4517, 6.45) ccw
  arc A314 (29.9314, -2.3471) -> (30.9199, -2.0201) centre (26.7862, 8.8179) ccw
  arc A315 (28.7472, 0.3992) -> (29.2813, 0.5381) centre (27.304, 7.046) ccw
  arc A316 (29.2813, 0.5381) -> (30.0128, 0.7944) centre (26.6271, 9.2841) ccw
  arc A317 (30.0128, 0.7944) -> (30.9617, 1.223) centre (25.7177, 11.5695) ccw
  arc A318 (28.548, 3.4019) -> (29.0646, 3.5959) centre (26.4179, 9.8615) ccw
  arc A319 (29.0646, 3.5959) -> (29.7653, 3.9273) centre (25.5108, 12.0165) ccw
  arc A320 (29.7653, 3.9273) -> (30.6643, 4.4527) centre (24.3675, 14.1944) ccw
  arc A321 (28.036, 6.3674) -> (28.5295, 6.6143) centre (25.2424, 12.5689) ccw
  arc A322 (28.5295, 6.6143) -> (29.1918, 7.0171) centre (24.1149, 14.6173) ccw
  arc A323 (29.1918, 7.0171) -> (30.0309, 7.6336) centre (22.7503, 16.6637) ccw
  arc A324 (27.2169, 9.2631) -> (27.6819, 9.5602) centre (23.7903, 15.1386) ccw
  arc A325 (27.6819, 9.5602) -> (28.2984, 10.03) centre (22.4549, 17.0579) ccw
  arc A326 (28.2984, 10.03) -> (29.0684, 10.7308) centre (20.8838, 18.9505) ccw
  arc A327 (26.0995, 12.0573) -> (26.5309, 12.4013) centre (22.0776, 17.5424) ccw
  arc A328 (26.5309, 12.4013) -> (27.0949, 12.933) centre (20.5489, 19.3117) ccw
  arc A329 (27.0949, 12.933) -> (27.7875, 13.7105) centre (18.7885, 21.0296) ccw
  arc A330 (24.6962, 14.7194) -> (25.0893, 15.1066) centre (20.123, 19.754) ccw
  arc A331 (25.0893, 15.1066) -> (25.5946, 15.6944) centre (18.4177, 21.3538) ccw
  arc A332 (25.5946, 15.6944) -> (26.2021, 16.54) centre (16.4874, 22.8784) ccw
  arc A333 (23.0223, 17.2202) -> (23.3728, 17.6464) centre (17.9479, 21.7493) ccw
  arc A334 (23.3728, 17.6464) -> (23.8139, 18.2838) centre (16.0847, 23.162) ccw
  arc A335 (23.8139, 18.2838) -> (24.3297, 19.1883) centre (14.0056, 24.4764) ccw
  arc A336 (21.0962, 19.5323) -> (21.4002, 19.9929) centre (15.5761, 23.5062) ccw
  arc A337 (21.4002, 19.9929) -> (21.7723, 20.6728) centre (13.5755, 24.7164) ccw
  arc A338 (21.7723, 20.6728) -> (22.1907, 21.6263) centre (11.3704, 25.8063) ccw
  arc A339 (18.939, 21.6305) -> (19.1931, 22.1203) centre (13.0337, 25.0056) ccw
  arc A340 (19.1931, 22.1203) -> (19.4921, 22.8354) centre (10.9176, 26.0001) ccw
  arc A341 (19.4921, 22.8354) -> (19.8086, 23.8274) centre (8.6106, 26.8535) ccw
  arc A342 (16.5742, 23.4917) -> (16.7758, 24.0053) centre (10.3486, 26.231) ccw
  arc A343 (16.7758, 24.0053) -> (16.9984, 24.7478) centre (8.14, 26.9988) ccw
  arc A344 (16.9984, 24.7478) -> (17.2094, 25.7674) centre (5.7565, 27.6065) ccw
  arc A345 (14.0279, 25.0954) -> (14.1746, 25.6274) centre (7.55, 27.169) ccw
  arc A346 (14.1746, 25.6274) -> (14.3184, 26.389) centre (5.2733, 27.7018) ccw
  arc A347 (14.3184, 26.389) -> (14.4217, 27.4251) centre (2.8393, 28.057) ccw
  arc A348 (11.3278, 26.4243) -> (11.4182, 26.9686) centre (4.6687, 27.8093) ccw
  arc A349 (11.4182, 26.9686) -> (11.4816, 27.7412) centre (2.3488, 28.1012) ccw
  arc A350 (11.4816, 27.7412) -> (11.476, 28.7824) centre (-0.109, 28.2) ccw
  arc A351 (8.5037, 27.4636) -> (8.5367, 28.0144) centre (1.7362, 28.145) ccw
  arc A352 (8.5367, 28.0144) -> (8.5189, 28.7893) centre (-0.6015, 28.1928) ccw
  arc A353 (8.5189, 28.7893) -> (8.4046, 29.8243) centre (-3.0561, 28.0342) ccw
  arc A354 (5.5864, 28.202) -> (5.5616, 28.7533) centre (-1.2152, 28.1723) ccw
  arc A355 (5.5616, 28.7533) -> (5.4629, 29.5221) centre (-3.5452, 27.9755) ccw
  arc A356 (5.4629, 29.5221) -> (5.241, 30.5394) centre (-5.9697, 27.5611) ccw
  arc A357 (2.6079, 28.6315) -> (2.5256, 29.1771) centre (-4.1534, 27.891) ccw
  arc A358 (2.5256, 29.1771) -> (2.3471, 29.9314) centre (-6.45, 27.4517) ccw
  arc A359 (2.3471, 29.9314) -> (2.0201, 30.9199) centre (-8.8179, 26.7862) ccw
  arc A360 (0.3992, 28.7472) -> (-0.3992, 28.7472) centre (0, 0) ccw
  arc A361 (-2.6079, 28.6315) -> (-3.4019, 28.548) centre (0, 0) ccw
  arc A362 (-5.5864, 28.202) -> (-6.3674, 28.036) centre (0, 0) ccw
  arc A363 (-8.5037, 27.4636) -> (-9.2631, 27.2169) centre (0, 0) ccw
  arc A364 (-11.3278, 26.4243) -> (-12.0573, 26.0995) centre (0, 0) ccw
  arc A365 (-14.0279, 25.0954) -> (-14.7194, 24.6962) centre (0, 0) ccw
  arc A366 (-16.5742, 23.4917) -> (-17.2202, 23.0223) centre (0, 0) ccw
  arc A367 (-18.939, 21.6305) -> (-19.5323, 21.0962) centre (0, 0) ccw
  arc A368 (-21.0962, 19.5323) -> (-21.6305, 18.939) centre (0, 0) ccw
  arc A369 (-23.0223, 17.2202) -> (-23.4917, 16.5742) centre (0, 0) ccw
  arc A370 (-24.6962, 14.7194) -> (-25.0954, 14.0279) centre (0, 0) ccw
  arc A371 (-26.0995, 12.0573) -> (-26.4243, 11.3278) centre (0, 0) ccw
  arc A372 (-27.2169, 9.2631) -> (-27.4636, 8.5037) centre (0, 0) ccw
  arc A373 (-28.036, 6.3674) -> (-28.202, 5.5864) centre (0, 0) ccw
  arc A374 (-28.548, 3.4019) -> (-28.6315, 2.6079) centre (0, 0) ccw
  arc A375 (-28.7472, 0.3992) -> (-28.7472, -0.3992) centre (0, 0) ccw
  arc A376 (-28.6315, -2.6079) -> (-28.548, -3.4019) centre (0, 0) ccw
  arc A377 (-28.202, -5.5864) -> (-28.036, -6.3674) centre (0, 0) ccw
  arc A378 (-27.4636, -8.5037) -> (-27.2169, -9.2631) centre (0, 0) ccw
  arc A379 (-26.4243, -11.3278) -> (-26.0995, -12.0573) centre (0, 0) ccw
  arc A380 (-25.0954, -14.0279) -> (-24.6962, -14.7194) centre (0, 0) ccw
  arc A381 (-23.4917, -16.5742) -> (-23.0223, -17.2202) centre (0, 0) ccw
  arc A382 (-21.6305, -18.939) -> (-21.0962, -19.5323) centre (0, 0) ccw
  arc A383 (-19.5323, -21.0962) -> (-18.939, -21.6305) centre (0, 0) ccw
  arc A384 (-17.2202, -23.0223) -> (-16.5742, -23.4917) centre (0, 0) ccw
  arc A385 (-14.7194, -24.6962) -> (-14.0279, -25.0954) centre (0, 0) ccw
  arc A386 (-12.0573, -26.0995) -> (-11.3278, -26.4243) centre (0, 0) ccw
  arc A387 (-9.2631, -27.2169) -> (-8.5037, -27.4636) centre (0, 0) ccw
  arc A388 (-6.3674, -28.036) -> (-5.5864, -28.202) centre (0, 0) ccw
  arc A389 (-3.4019, -28.548) -> (-2.6079, -28.6315) centre (0, 0) ccw
  arc A390 (-0.3992, -28.7472) -> (0.3992, -28.7472) centre (0, 0) ccw
  arc A391 (2.6079, -28.6315) -> (3.4019, -28.548) centre (0, 0) ccw
  arc A392 (5.5864, -28.202) -> (6.3674, -28.036) centre (0, 0) ccw
  arc A393 (8.5037, -27.4636) -> (9.2631, -27.2169) centre (0, 0) ccw
  arc A394 (11.3278, -26.4243) -> (12.0573, -26.0995) centre (0, 0) ccw
  arc A395 (14.0279, -25.0954) -> (14.7194, -24.6962) centre (0, 0) ccw
  arc A396 (16.5742, -23.4917) -> (17.2202, -23.0223) centre (0, 0) ccw
  arc A397 (18.939, -21.6305) -> (19.5323, -21.0962) centre (0, 0) ccw
  arc A398 (21.0962, -19.5323) -> (21.6305, -18.939) centre (0, 0) ccw
  arc A399 (23.0223, -17.2202) -> (23.4917, -16.5742) centre (0, 0) ccw
  arc A400 (24.6962, -14.7194) -> (25.0954, -14.0279) centre (0, 0) ccw
  arc A401 (26.0995, -12.0573) -> (26.4243, -11.3278) centre (0, 0) ccw
  arc A402 (27.2169, -9.2631) -> (27.4636, -8.5037) centre (0, 0) ccw
  arc A403 (28.036, -6.3674) -> (28.202, -5.5864) centre (0, 0) ccw
  arc A404 (28.548, -3.4019) -> (28.6315, -2.6079) centre (0, 0) ccw
  arc A405 (28.7472, -0.3992) -> (28.7472, 0.3992) centre (0, 0) ccw
  arc A406 (28.6315, 2.6079) -> (28.548, 3.4019) centre (0, 0) ccw
  arc A407 (28.202, 5.5864) -> (28.036, 6.3674) centre (0, 0) ccw
  arc A408 (27.4636, 8.5037) -> (27.2169, 9.2631) centre (0, 0) ccw
  arc A409 (26.4243, 11.3278) -> (26.0995, 12.0573) centre (0, 0) ccw
  arc A410 (25.0954, 14.0279) -> (24.6962, 14.7194) centre (0, 0) ccw
  arc A411 (23.4917, 16.5742) -> (23.0223, 17.2202) centre (0, 0) ccw
  arc A412 (21.6305, 18.939) -> (21.0962, 19.5323) centre (0, 0) ccw
  arc A413 (19.5323, 21.0962) -> (18.939, 21.6305) centre (0, 0) ccw
  arc A414 (17.2202, 23.0223) -> (16.5742, 23.4917) centre (0, 0) ccw
  arc A415 (14.7194, 24.6962) -> (14.0279, 25.0954) centre (0, 0) ccw
  arc A416 (12.0573, 26.0995) -> (11.3278, 26.4243) centre (0, 0) ccw
  arc A417 (9.2631, 27.2169) -> (8.5037, 27.4636) centre (0, 0) ccw
  arc A418 (6.3674, 28.036) -> (5.5864, 28.202) centre (0, 0) ccw
  arc A419 (3.4019, 28.548) -> (2.6079, 28.6315) centre (0, 0) ccw
  arc A420 (-1.223, 30.9617) -> (-2.0201, 30.9199) centre (0, 0) ccw
  arc A421 (-4.4527, 30.6643) -> (-5.241, 30.5394) centre (0, 0) ccw
  arc A422 (-7.6336, 30.0309) -> (-8.4046, 29.8243) centre (0, 0) ccw
  arc A423 (-10.7308, 29.0684) -> (-11.476, 28.7824) centre (0, 0) ccw
  arc A424 (-13.7105, 27.7875) -> (-14.4217, 27.4251) centre (0, 0) ccw
  arc A425 (-16.54, 26.2021) -> (-17.2094, 25.7674) centre (0, 0) ccw
  arc A426 (-19.1883, 24.3297) -> (-19.8086, 23.8274) centre (0, 0) ccw
  arc A427 (-21.6263, 22.1907) -> (-22.1907, 21.6263) centre (0, 0) ccw
  arc A428 (-23.8274, 19.8086) -> (-24.3297, 19.1883) centre (0, 0) ccw
  arc A429 (-25.7674, 17.2094) -> (-26.2021, 16.54) centre (0, 0) ccw
  arc A430 (-27.4251, 14.4217) -> (-27.7875, 13.7105) centre (0, 0) ccw
  arc A431 (-28.7824, 11.476) -> (-29.0684, 10.7308) centre (0, 0) ccw
  arc A432 (-29.8243, 8.4046) -> (-30.0309, 7.6336) centre (0, 0) ccw
  arc A433 (-30.5394, 5.241) -> (-30.6643, 4.4527) centre (0, 0) ccw
  arc A434 (-30.9199, 2.0201) -> (-30.9617, 1.223) centre (0, 0) ccw
  arc A435 (-30.9617, -1.223) -> (-30.9199, -2.0201) centre (0, 0) ccw
  arc A436 (-30.6643, -4.4527) -> (-30.5394, -5.241) centre (0, 0) ccw
  arc A437 (-30.0309, -7.6336) -> (-29.8243, -8.4046) centre (0, 0) ccw
  arc A438 (-29.0684, -10.7308) -> (-28.7824, -11.476) centre (0, 0) ccw
  arc A439 (-27.7875, -13.7105) -> (-27.4251, -14.4217) centre (0, 0) ccw
  arc A440 (-26.2021, -16.54) -> (-25.7674, -17.2094) centre (0, 0) ccw
  arc A441 (-24.3297, -19.1883) -> (-23.8274, -19.8086) centre (0, 0) ccw
  arc A442 (-22.1907, -21.6263) -> (-21.6263, -22.1907) centre (0, 0) ccw
  arc A443 (-19.8086, -23.8274) -> (-19.1883, -24.3297) centre (0, 0) ccw
  arc A444 (-17.2094, -25.7674) -> (-16.54, -26.2021) centre (0, 0) ccw
  arc A445 (-14.4217, -27.4251) -> (-13.7105, -27.7875) centre (0, 0) ccw
  arc A446 (-11.476, -28.7824) -> (-10.7308, -29.0684) centre (0, 0) ccw
  arc A447 (-8.4046, -29.8243) -> (-7.6336, -30.0309) centre (0, 0) ccw
  arc A448 (-5.241, -30.5394) -> (-4.4527, -30.6643) centre (0, 0) ccw
  arc A449 (-2.0201, -30.9199) -> (-1.223, -30.9617) centre (0, 0) ccw
  arc A450 (1.223, -30.9617) -> (2.0201, -30.9199) centre (0, 0) ccw
  arc A451 (4.4527, -30.6643) -> (5.241, -30.5394) centre (0, 0) ccw
  arc A452 (7.6336, -30.0309) -> (8.4046, -29.8243) centre (0, 0) ccw
  arc A453 (10.7308, -29.0684) -> (11.476, -28.7824) centre (0, 0) ccw
  arc A454 (13.7105, -27.7875) -> (14.4217, -27.4251) centre (0, 0) ccw
  arc A455 (16.54, -26.2021) -> (17.2094, -25.7674) centre (0, 0) ccw
  arc A456 (19.1883, -24.3297) -> (19.8086, -23.8274) centre (0, 0) ccw
  arc A457 (21.6263, -22.1907) -> (22.1907, -21.6263) centre (0, 0) ccw
  arc A458 (23.8274, -19.8086) -> (24.3297, -19.1883) centre (0, 0) ccw
  arc A459 (25.7674, -17.2094) -> (26.2021, -16.54) centre (0, 0) ccw
  arc A460 (27.4251, -14.4217) -> (27.7875, -13.7105) centre (0, 0) ccw
  arc A461 (28.7824, -11.476) -> (29.0684, -10.7308) centre (0, 0) ccw
  arc A462 (29.8243, -8.4046) -> (30.0309, -7.6336) centre (0, 0) ccw
  arc A463 (30.5394, -5.241) -> (30.6643, -4.4527) centre (0, 0) ccw
  arc A464 (30.9199, -2.0201) -> (30.9617, -1.223) centre (0, 0) ccw
  arc A465 (30.9617, 1.223) -> (30.9199, 2.0201) centre (0, 0) ccw
  arc A466 (30.6643, 4.4527) -> (30.5394, 5.241) centre (0, 0) ccw
  arc A467 (30.0309, 7.6336) -> (29.8243, 8.4046) centre (0, 0) ccw
  arc A468 (29.0684, 10.7308) -> (28.7824, 11.476) centre (0, 0) ccw
  arc A469 (27.7875, 13.7105) -> (27.4251, 14.4217) centre (0, 0) ccw
  arc A470 (26.2021, 16.54) -> (25.7674, 17.2094) centre (0, 0) ccw
  arc A471 (24.3297, 19.1883) -> (23.8274, 19.8086) centre (0, 0) ccw
  arc A472 (22.1907, 21.6263) -> (21.6263, 22.1907) centre (0, 0) ccw
  arc A473 (19.8086, 23.8274) -> (19.1883, 24.3297) centre (0, 0) ccw
  arc A474 (17.2094, 25.7674) -> (16.54, 26.2021) centre (0, 0) ccw
  arc A475 (14.4217, 27.4251) -> (13.7105, 27.7875) centre (0, 0) ccw
  arc A476 (11.476, 28.7824) -> (10.7308, 29.0684) centre (0, 0) ccw
  arc A477 (8.4046, 29.8243) -> (7.6336, 30.0309) centre (0, 0) ccw
  arc A478 (5.241, 30.5394) -> (4.4527, 30.6643) centre (0, 0) ccw
  arc A479 (2.0201, 30.9199) -> (1.223, 30.9617) centre (0, 0) ccw
  point P0 (0, 0)
  constraints: 720 point on circle, 360 centre point, 2 horizontal alignment, 2 vertical alignment, 356 other
extrude "Extrusion1" add sketch "Sketch1" against normal blind 4
body "Solid1"
